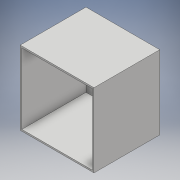
# Autodesk Inventor part: UltimakerDruckgroesse_MAX
Saved by Autodesk Inventor 2017 (Build 210142000, 142)
## iProperties
Created: 2019-05-23
Part Number: UltimakerDruckgroesse_MAX
Material: Generic
Document SubType Name: Modeling
Designer: Ole Simmering
Density: 1 g/cm^3
Appearance: Default
Author: Ole Simmering
Autodesk Inventor part; units mm, degrees
ref_plane "YZ Plane" through (0, 0, 0) normal (1, 0, 0) x (0, 1, 0)
ref_plane "XZ Plane" through (0, 0, 0) normal (0, 1, 0) x (-1, 0, 0)
ref_plane "XY Plane" through (0, 0, 0) normal (0, 0, 1) x (1, 0, 0)
sketch "Sketch1" plane through (0, 0, 0) normal (0, 1, 0) x (-1, 0, 0)
  line L0 (0, 0) -> (-221, 0)
  line L1 (-221, 0) -> (-221, 221)
  line L2 (-221, 221) -> (0, 221)
  line L3 (0, 221) -> (0, 0)
  line L4 (5, -5) -> (-226, -5)
  line L5 (-226, -5) -> (-226, 226)
  line L6 (-226, 226) -> (5, 226)
  line L7 (5, 226) -> (5, -5)
  dimension "d0" = 221
  dimension "d1" = 221
  dimension "d2" = 5
  constraints: 16 end point, 4 parallel, 2 perpendicular, 1 horizontal, 3 other
  measures "d0" distance of L1.end L2.end
  measures "d1" distance of L0.end L1.end
  measures "d2" distance between parallel lines of L3 L7
extrude "Extrusion1" add sketch "Sketch1" along normal blind 201
sketch "Sketch2" plane through (0, 201, 0) normal (0, 1, 0) x (1, 0, 0)
  line L0 (226, 5) -> (226, -226) projected
  line L1 (-5, -226) -> (226, -226)
  line L2 (226, -226) -> (226, 5)
  line L3 (226, 5) -> (-5, 5)
  line L4 (-5, 5) -> (-5, -226)
  point P0 (0, 0)
  constraints: 8 end point, 2 parallel, 1 horizontal, 1 perpendicular
extrude "Extrusion2" add sketch "Sketch2" along normal blind 5
body "Solid1"
